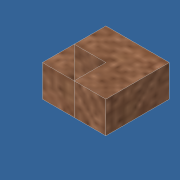
# Autodesk Inventor part: Brown Part
Saved by Autodesk Inventor 2018 (Build 220112000, 112)
## iProperties
Created: 2017-11-14
Part Number: Brown Part
Material: Wood (Maple)
Document SubType Name: Modeling
Designer: 232963
Density: 0.67 g/cm^3
Appearance: Brown
Author: 232963
Autodesk Inventor part; units mm, degrees
ref_plane "YZ Plane" through (0, 0, 0) normal (1, 0, 0) x (0, 1, 0)
ref_plane "XZ Plane" through (0, 0, 0) normal (0, 1, 0) x (-1, 0, 0)
ref_plane "XY Plane" through (0, 0, 0) normal (0, 0, 1) x (1, 0, 0)
sketch "Sketch1" plane through (0, 0, 0) normal (0, 0, 1) x (1, 0, 0)
  line L0 (-15.0104, -7.0026) -> (23.0896, -7.0026)
  line L1 (23.0896, -7.0026) -> (23.0896, 5.0447)
  line L2 (4.0396, 12.0474) -> (-15.0104, 12.0474)
  line L3 (-15.0104, 12.0474) -> (-15.0104, -7.0026)
  line L4 (23.0896, -7.0026) -> (4.0396, -7.0026)
  line L5 (4.0396, 12.0474) -> (4.0396, 31.0974)
  line L6 (4.0396, 31.0974) -> (23.0896, 31.0974)
  line L7 (23.0896, 31.0974) -> (23.0896, -7.0026)
  point P0 (0, 0)
  dimension "d0" = 19.05
  dimension "d1" = 19.05
  dimension "d2" = 19.05
  dimension "d3" = 38.1
  constraints: 16 end point, 4 parallel, 2 horizontal, 2 perpendicular
  measures "d0" distance of L2.start L2.end
  measures "d1" distance of L2.end L0.start
  measures "d2" distance of L5.end L6.end
  measures "d3" distance of L6.end L0.end
extrude "Extrusion1" add sketch "Sketch1" along normal blind 19.05
sketch "Sketch2" plane through (23.0896, -7.0026, 0) normal (1, 0, 0) x (0, 0, -1)
  line L0 (0, 38.1) -> (-19.05, 38.1) projected
  line L1 (0, 38.1) -> (-38.1, 38.1)
  line L2 (-38.1, 38.1) -> (-38.1, 19.05)
  line L3 (-38.1, 19.05) -> (0, 19.05)
  line L4 (0, 19.05) -> (0, 38.1)
  point P0 (0, 7.0026)
  dimension "d6" = 38.1
  dimension "d7" = 19.05
  constraints: 8 end point, 2 parallel, 1 horizontal, 1 perpendicular
  measures "d6" distance of L2.end L3.end
  measures "d7" distance of L1.end L2.end
extrude "Extrusion2" add sketch "Sketch2" along normal blind 19.05
body "Solid1"
